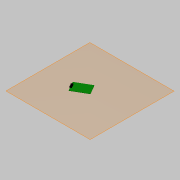
# Autodesk Inventor part: Part1
Saved by Autodesk Inventor 2014 (Build 180170000, 170)
## iProperties
Created: 2016-03-30
Part Number: Part1
Material: Aluminum 6061
Document SubType Name: Modeling
Designer: admin
Density: 2.71 g/cm^3
Appearance: Dark Green
Author: admin
Autodesk Inventor part; units mm, degrees
ref_plane "YZ Plane" through (0, 0, 0) normal (1, 0, 0) x (0, 1, 0)
ref_plane "XZ Plane" through (0, 0, 0) normal (0, 1, 0) x (-1, 0, 0)
ref_plane "XY Plane" through (0, 0, 0) normal (0, 0, 1) x (1, 0, 0)
ref_plane "Work Plane1" through (0, 0, 0) normal (0, 0, 1) x (1, 0, 0)
sketch "Sketch1" plane through (0, 0, 0) normal (0, 0, 1) x (1, 0, 0)
  line L0 (-106.8732, -139.6455) -> (-150.8241, -63.5202) projected
  line L1 (-148.3027, -27.8876) -> (-98.3027, -114.4901)
  line L2 (-98.3027, -114.4901) -> (27.271, -41.9901)
  line L3 (27.271, -41.9901) -> (-22.729, 44.6124)
  line L4 (-22.729, 44.6124) -> (-148.3027, -27.8876)
  line L5 (-174.3732, -22.7321) -> (-171.7751, -21.2321) projected
  line L6 (-123.3027, -71.1888) -> (2.271, 1.3112)
  circle A0 centre (-141.4725, -29.7177) radius 1.5
  circle A1 centre (-96.4725, -107.66) radius 1.5
  circle A2 centre (-24.5591, 37.7823) radius 1.5
  circle A3 centre (20.4409, -40.16) radius 1.5
  line L7 (-106.4027, -100.4605) -> (19.171, -27.9605)
  line L8 (-117.6027, -81.0615) -> (7.971, -8.5615)
  line L9 (-126.7027, -65.2999) -> (-1.129, 7.2001)
  dimension "d3" = 100
  dimension "d4" = 145
  dimension "d5" = 67.5
  dimension "d6" = 20
  dimension "d7" = 3
  dimension "d8" = 3
  dimension "d9" = 3
  dimension "d10" = 3
  dimension "d11" = 5
  dimension "d12" = 5
  dimension "d13" = 5
  dimension "d14" = 5
  dimension "d15" = 5
  dimension "d16" = 5
  dimension "d17" = 5
  dimension "d18" = 5
  dimension "d19" = 16.2
  dimension "d20" = 38.6
  dimension "d21" = 56.8
  constraints: 16 end point, 6 point on line, 4 centre point, 4 perpendicular, 3 parallel, 2 midpoint
  measures "d3" distance of L1.start L1.end
  measures "d4" distance of L2.end L1.end
  measures "d5" distance between parallel lines of L5 L6
  measures "d6" distance between parallel lines of L0 L1
  measures "d7" diameter of A0
  measures "d8" diameter of A1
  measures "d9" diameter of A2
  measures "d10" diameter of A3
  measures "d11" distance from line of L4 A0.centre
  measures "d12" distance from line of L1 A0.centre
  measures "d13" distance from line of L2 A1.centre
  measures "d14" distance from line of L1 A1.centre
  measures "d15" distance from line of L3 A3.centre
  measures "d16" distance from line of L2 A3.centre
  measures "d17" distance from line of L3 A2.centre
  measures "d18" distance from line of L4 A2.centre
  measures "d19" distance between parallel lines of L2 L7
  measures "d20" distance between parallel lines of L2 L8
  measures "d21" distance between parallel lines of L9 L2
extrude "Extrusion1" add sketch "Sketch1" along normal blind 1.8
sketch "Sketch2" plane through (0, 0, 1.8) normal (0, 0, 1) x (1, 0, 0)
  line L0 (27.271, -41.9901) -> (-22.729, 44.6124) projected
  line L1 (-148.3027, -27.8876) -> (-98.3027, -114.4901) projected
  line L2 (-98.3027, -114.4901) -> (27.271, -41.9901) projected
  line L3 (-106.4027, -100.4605) -> (19.171, -27.9605)
  line L4 (-117.6027, -81.0615) -> (7.971, -8.5615)
  line L5 (-1.129, 7.2001) -> (-126.7027, -65.2999)
  line L6 (-130.7027, -58.3717) -> (-122.7027, -72.2281)
  line L7 (-122.7027, -72.2281) -> (-110.2319, -65.0281)
  line L8 (-110.2319, -65.0281) -> (-118.2319, -51.1717)
  line L9 (-118.2319, -51.1717) -> (-130.7027, -58.3717)
  line L10 (-120.6527, -75.7788) -> (-114.5527, -86.3443)
  line L11 (-114.5527, -86.3443) -> (-102.8613, -79.5943)
  line L12 (-102.8613, -79.5943) -> (-108.9613, -69.0288)
  line L13 (-108.9613, -69.0288) -> (-120.6527, -75.7788)
  line L14 (-111.0027, -92.4931) -> (-101.8027, -108.4279)
  line L15 (-101.8027, -108.4279) -> (-86.7338, -99.7279)
  line L16 (-86.7338, -99.7279) -> (-95.9338, -83.7931)
  line L17 (-95.9338, -83.7931) -> (-111.0027, -92.4931)
  line L18 (-251.5686, 33.0808) -> (-251.5686, 18.7808)
  line L19 (-253.5686, -22.5192) -> (-253.5686, -6.8192)
  line L20 (-249.5686, -8.2192) -> (-249.5686, -21.1192)
  line L21 (-462.5686, 42.1808) -> (-462.5686, -97.8192)
  line L22 (-412.5686, -27.8192) -> (-252.5686, -27.8192)
  line L23 (-269.9686, 33.0808) -> (-251.5686, 33.0808)
  line L24 (-252.5686, -26.8192) -> (-412.5686, -26.8192)
  line L25 (-249.5686, 36.4808) -> (-251.5686, 36.4808)
  line L26 (-251.5686, 15.3808) -> (-249.5686, 15.3808)
  line L27 (-252.5686, -27.8192) -> (-252.5686, -97.8192)
  line L28 (-462.5686, -97.8192) -> (-252.5686, -97.8192)
  line L29 (-252.5686, 32.3808) -> (-252.5686, 18.0808)
  line L30 (-249.5686, 15.3808) -> (-249.5686, 36.4808)
  line L31 (-266.9686, -6.8192) -> (-266.9686, -22.5192)
  line L32 (-253.5686, -21.1192) -> (-253.5686, -8.2192)
  line L33 (-249.5686, 9.6808) -> (-249.5686, -2.5192)
  line L34 (-252.5686, 42.1808) -> (-462.5686, 42.1808)
  line L35 (-246.5575, 29.6636) -> (-249.5686, 18.6388)
  line L36 (-252.5686, -8.2192) -> (-252.5686, -21.1192)
  circle A0 centre (-257.5686, 37.1808) radius 2.5
  line L37 (-251.5686, 18.7808) -> (-269.9686, 18.7808)
  line L38 (-251.5686, 36.4808) -> (-251.5686, 15.3808)
  line L39 (-266.9686, -22.5192) -> (-253.5686, -22.5192)
  line L40 (-249.5686, -21.1192) -> (-253.5686, -21.1192)
  circle A1 centre (-257.5686, 37.1808) radius 1.5
  line L41 (-252.5686, 42.1808) -> (-412.5686, 42.1808)
  line L42 (-249.5686, 33.0078) -> (-246.5575, 29.6636)
  line L43 (-252.5686, -27.8192) -> (-252.5686, 42.1808)
  circle A2 centre (-257.5686, 37.1808) radius 2.5
  line L44 (-269.9686, 18.7808) -> (-269.9686, 33.0808)
  line L45 (-266.0686, -2.5192) -> (-266.0686, 9.6808)
  line L46 (-412.5686, 42.1808) -> (-412.5686, -27.8192)
  line L47 (-252.5686, -21.1192) -> (-252.5686, -8.2192)
  line L48 (-266.0686, 9.6808) -> (-249.5686, 9.6808)
  line L49 (-253.5686, -6.8192) -> (-266.9686, -6.8192)
  line L50 (-249.5686, -2.5192) -> (-266.0686, -2.5192)
  line L51 (-253.5686, -8.2192) -> (-249.5686, -8.2192)
  line L52 (-249.5686, -8.2192) -> (-252.5686, -8.2192)
  line L53 (-252.5686, -21.1192) -> (-249.5686, -21.1192)
  line L54 (-249.5686, -21.1192) -> (-249.5686, -8.2192)
  line L55 (-252.5686, -2.5192) -> (-249.5686, -2.5192)
  line L56 (-249.5686, 9.6808) -> (-252.5686, 9.6808)
  line L57 (-249.5686, 18.6388) -> (-246.5575, 29.6636)
  line L58 (-249.5686, -2.5192) -> (-249.5686, 9.6808)
  line L59 (-246.5575, 29.6636) -> (-249.5686, 33.0078)
  line L60 (-246.5575, 29.6636) -> (-249.5686, 33.0078)
  line L61 (-249.5686, 33.0078) -> (-249.5686, 18.6388)
  line L62 (-249.5686, 18.6388) -> (-246.5575, 29.6636)
  line L63 (-249.5686, 33.0078) -> (-249.5686, 18.6388)
  line L64 (-252.5686, -21.1192) -> (-252.5686, -8.2192)
  line L65 (-249.5686, 36.4808) -> (-251.5686, 36.4808)
  line L66 (-462.5686, -97.8192) -> (-252.5686, -97.8192)
  line L67 (-251.5686, 15.3808) -> (-249.5686, 15.3808)
  line L68 (-251.5686, 18.7808) -> (-251.5686, 15.3808)
  line L69 (-252.5686, 18.7808) -> (-251.5686, 18.7808)
  line L70 (-251.5686, 33.0808) -> (-252.5686, 33.0808)
  line L71 (-251.5686, 36.4808) -> (-251.5686, 33.0808)
  line L72 (-249.5686, 15.3808) -> (-249.5686, 36.4808)
  line L73 (-462.5686, -97.8192) -> (-462.5686, 42.1808)
  line L74 (-462.5686, 42.1808) -> (-462.5686, -97.8192)
  line L75 (-252.5686, 18.7808) -> (-252.5686, -97.8192)
  line L76 (-252.5686, 42.1808) -> (-252.5686, 33.0808)
  line L77 (-252.5686, -97.8192) -> (-252.5686, 42.1808)
  line L78 (-252.5686, 9.6808) -> (-252.5686, -2.5192)
  line L79 (-252.5686, -97.8192) -> (-462.5686, -97.8192)
  line L80 (-462.5686, 42.1808) -> (-252.5686, 42.1808)
  line L81 (-252.5686, 42.1808) -> (-462.5686, 42.1808)
  line L82 (-252.5686, 18.7808) -> (-251.5686, 18.7808)
  line L83 (-249.5686, -2.5192) -> (-249.5686, 9.6808)
  line L84 (-249.5686, 9.6808) -> (-252.5686, 9.6808)
  line L85 (-252.5686, -2.5192) -> (-249.5686, -2.5192)
  line L86 (-251.5686, 36.4808) -> (-251.5686, 33.0808)
  line L87 (-251.5686, 33.0808) -> (-252.5686, 33.0808)
  line L88 (-252.5686, 18.7808) -> (-252.5686, 33.0808)
  line L89 (-251.5686, 18.7808) -> (-251.5686, 15.3808)
  line L90 (-251.5686, 15.3808) -> (-249.5686, 15.3808)
  line L91 (-249.5686, 15.3808) -> (-249.5686, 36.4808)
  line L92 (-249.5686, 36.4808) -> (-251.5686, 36.4808)
  line L93 (-252.5686, -2.5192) -> (-252.5686, 9.6808)
  point P0 (0, 0)
  dimension "d24" = 16.2
  dimension "d25" = 38.6
  dimension "d26" = 56.8
  dimension "d27" = 14.4
  dimension "d28" = 13.5
  dimension "d29" = 17.4
  dimension "d30" = 9.2
  dimension "d31" = 9.2
  dimension "d32" = 6.1
  dimension "d33" = 6.1
  dimension "d34" = 8
  dimension "d35" = 8
  constraints: 182 end point, 6 parallel, 5 perpendicular, 3 centre point, 3 point on line, 11 other
  measures "d24" distance between parallel lines of L2 L3
  measures "d25" distance between parallel lines of L2 L4
  measures "d26" distance between parallel lines of L2 L5
  measures "d27" distance of L7.end L6.end
  measures "d28" distance of L11.end L10.end
  measures "d29" distance of L15.end L14.end
  measures "d30" distance between parallel lines of L3 L17
  measures "d31" distance between parallel lines of L15 L3
  measures "d32" distance between parallel lines of L4 L13
  measures "d33" distance between parallel lines of L11 L4
  measures "d34" distance between parallel lines of L5 L9
  measures "d35" distance between parallel lines of L7 L5
extrude "Extrusion2" add sketch "Sketch2" along normal blind 10.5 separate body contours L12 L11 L1 L4 | L4 L1 L13 L12 | L8 L7 L1 L5 | L5 L1 L9 L8
sketch "Sketch3" plane through (0, 0, 12.3) normal (0, 0, 1) x (1, 0, 0)
  line L0 (-122.7027, -72.2281) -> (-110.2319, -65.0281) projected
  line L1 (-110.2319, -65.0281) -> (-118.2319, -51.1717) projected
  line L2 (-118.2319, -51.1717) -> (-130.7027, -58.3717) projected
  line L3 (-130.7027, -58.3717) -> (-122.7027, -72.2281) projected
  point P0 (0, 0)
extrude "Extrusion3" add sketch "Sketch3" along normal blind 4 bodies 2
sketch "Sketch4" plane through (-122.7027, -72.2281, 1.8) normal (-0.866, -0.5, 0) x (0, 0, 1)
  circle A0 centre (7.25, 8) radius 6.5
  point P0 (-1.8, 1.2)
  dimension "d40" = 13
  constraints: 1 centre point
  measures "d40" diameter of A0
extrude "Extrusion4" add sketch "Sketch4" along normal blind 3 bodies 2
sketch "Sketch5" plane through (-114.5527, -86.3443, 1.8) normal (-0.866, -0.5, 0) x (0, 0, 1)
  line L0 (0, 12.2) -> (0, 0) projected
  line L1 (0, 0) -> (10.5, 0) projected
  line L2 (10.5, 12.2) -> (10.5, 0) projected
  line L3 (0, 12.2) -> (10.5, 12.2) projected
  point P0 (-1.8, 17.5)
extrude "Extrusion5" add sketch "Sketch5" along normal blind 3 bodies 2
sketch "Sketch6" plane through (-117.1507, -87.8443, 1.8) normal (-0.866, -0.5, 0) x (0, 0, 1)
  line L0 (0, 12.2) -> (0, 0) projected
  line L1 (0, 0) -> (10.5, 0) projected
  line L2 (10.5, 0) -> (10.5, 12.2) projected
  line L3 (10.5, 12.2) -> (0, 12.2) projected
  line L4 (1.5, 10.7) -> (1.5, 1.5)
  line L5 (1.5, 1.5) -> (9, 1.5)
  line L6 (9, 1.5) -> (9, 10.7)
  line L7 (9, 10.7) -> (1.5, 10.7)
  line L8 (4, 9) -> (7, 9)
  line L9 (7, 9) -> (7, 3)
  line L10 (7, 3) -> (4, 3)
  line L11 (4, 3) -> (4, 9)
  point P0 (-1.8, 17.5)
  dimension "d45" = 1.5
  constraints: 16 end point, 2 parallel, 1 horizontal, 1 perpendicular, 3 other
  measures "d45" distance between parallel lines of L3 L7
extrude "Extrusion6" cut sketch "Sketch6" against normal blind 10 contours L7 L6 L5 L4 bodies 2
chamfer "Chamfer1" distance 2 angle 45 2 edges at (-118.1698, -76.0773, 10.8) (-113.5698, -84.0447, 10.8)
sketch "Sketch11" plane through (-122.7027, -72.2281, 1.8) normal (-0.866, -0.5, 0) x (0, 0, 1)
  circle A0 centre (7.25, 8) radius 6.5 projected
  line L0 (0, 16) -> (0, 0) projected
  line L1 (0, 0) -> (14.5, 0) projected
  line L2 (14.5, 16) -> (14.5, 0) projected
  line L3 (0, 16) -> (14.5, 16) projected
  point P0 (-1.8, 1.2)
extrude "Extrusion11" cut sketch "Sketch11" against normal blind 1 bodies 2
body "Solid1"
body "Solid2"
